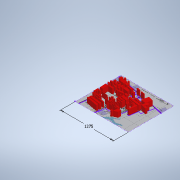
# Autodesk Inventor part: Ceg Model
Saved by Autodesk Inventor 2021 (Build 250183000, 183)
## iProperties
Created: 2021-08-03
Part Number: Ceg Model
Material: Generic
Document SubType Name: Modeling
Designer: techv
Density: 1 g/cm^3
Appearance: Default
Author: techv
Autodesk Inventor part; units mm, degrees
(part 1 of 2)
ref_plane "YZ Plane" through (0, 0, 0) normal (1, 0, 0) x (0, 1, 0)
ref_plane "XZ Plane" through (0, 0, 0) normal (0, 1, 0) x (-1, 0, 0)
ref_plane "XY Plane" through (0, 0, 0) normal (0, 0, 1) x (1, 0, 0)
sketch "Sketch1" plane through (0, 0, 0) normal (0, 1, 0) x (-1, 0, 0)
  line L0 (-1278471.3795, 0) -> (-3471.3795, 0) construction
  line L1 (-3471.3795, 0) -> (-3471.3795, -1090759.1919) construction
  line L2 (-3471.3795, -1090759.1919) -> (-1278471.3795, -1090759.1919) construction
  line L3 (-1278471.3795, -1090759.1919) -> (-1278471.3795, 0) construction
  line L4 (-570011.4545, -254930.8304) -> (-652781.9547, -243920.9646)
  line L5 (-652781.9547, -243920.9646) -> (-652781.9547, -234636.5388)
  line L6 (-652781.9547, -234636.5388) -> (-568797.9413, -245807.8223)
  line L7 (-568797.9413, -245807.8223) -> (-570011.4545, -254930.8304)
  line L8 (-501436.1788, -258320.5511) -> (-531092.2717, -254512.687)
  line L9 (-531092.2717, -254512.687) -> (-531551.829, -258091.7732)
  line L10 (-531551.829, -258091.7732) -> (-537674.5373, -257305.613)
  line L11 (-537674.5373, -257305.613) -> (-537674.5373, -262132.416)
  line L12 (-537674.5373, -262132.416) -> (-543243.6303, -262132.416)
  line L13 (-543243.6303, -262132.416) -> (-543243.6303, -255750.9615)
  line L14 (-543243.6303, -255750.9615) -> (-544918.8797, -255750.9615)
  line L15 (-544918.8797, -255750.9615) -> (-544918.8797, -248261.3499)
  line L16 (-544918.8797, -248261.3499) -> (-551485.4294, -248110.677)
  line L17 (-551485.4294, -248110.677) -> (-551473.9, -247608.2101)
  line L18 (-551473.9, -247608.2101) -> (-563231.7702, -247338.4195)
  line L19 (-563231.7702, -247338.4195) -> (-563178.5874, -245020.6323)
  line L20 (-563178.5874, -245020.6323) -> (-565590.3117, -244965.294)
  line L21 (-565590.3117, -244965.294) -> (-565542.041, -242861.5863)
  line L22 (-565542.041, -242861.5863) -> (-567752.7884, -242810.8595)
  line L23 (-567752.7884, -242810.8595) -> (-567622.1285, -237116.51)
  line L24 (-567622.1285, -237116.51) -> (-565411.3812, -237167.2367)
  line L25 (-565411.3812, -237167.2367) -> (-565358.3685, -234856.8655)
  line L26 (-565358.3685, -234856.8655) -> (-559798.004, -234984.451)
  line L27 (-559798.004, -234984.451) -> (-559904.8178, -239639.5544)
  line L28 (-559904.8178, -239639.5544) -> (-558119.111, -239680.5284)
  line L29 (-558119.111, -239680.5284) -> (-558038.8035, -236180.6106)
  line L30 (-558038.8035, -236180.6106) -> (-549698.723, -236371.9782)
  line L31 (-549698.723, -236371.9782) -> (-549769.374, -239451.0531)
  line L32 (-549769.374, -239451.0531) -> (-547223.665, -239509.4657)
  line L33 (-547223.665, -239509.4657) -> (-547179.5203, -237585.5765)
  line L34 (-547179.5203, -237585.5765) -> (-540070.8135, -237748.6895)
  line L35 (-540070.8135, -237748.6895) -> (-540175.7779, -242323.193)
  line L36 (-540175.7779, -242323.193) -> (-536543.1178, -242406.5463)
  line L37 (-536543.1178, -242406.5463) -> (-536455.3851, -238583.0282)
  line L38 (-536455.3851, -238583.0282) -> (-529068.6548, -238752.5206)
  line L39 (-529068.6548, -238752.5206) -> (-529283.5365, -248117.3798)
  line L40 (-529283.5365, -248117.3798) -> (-523156.9583, -248257.9574)
  line L41 (-523156.9583, -248257.9574) -> (-523160.4206, -248408.8486)
  line L42 (-523160.4206, -248408.8486) -> (-520279.7498, -248474.9471)
  line L43 (-520279.7498, -248474.9471) -> (-520276.2876, -248324.0559)
  line L44 (-520276.2876, -248324.0559) -> (-515159.0607, -248441.4734)
  line L45 (-515159.0607, -248441.4734) -> (-515162.523, -248592.3646)
  line L46 (-515162.523, -248592.3646) -> (-511493.6444, -248676.5489)
  line L47 (-511493.6444, -248676.5489) -> (-511460.6396, -247238.1505)
  line L48 (-511460.6396, -247238.1505) -> (-506111.3606, -247360.8925)
  line L49 (-506111.3606, -247360.8925) -> (-506184.1973, -250535.222)
  line L50 (-506184.1973, -250535.222) -> (-502834.5802, -250612.0808)
  line L51 (-502834.5802, -250612.0808) -> (-502802.8154, -249227.7254)
  line L52 (-502802.8154, -249227.7254) -> (-500231.0639, -248934.9748)
  line L53 (-500231.0639, -248934.9748) -> (-501436.1788, -258320.5511)
  line L54 (-576349.5369, -265725.8408) -> (-577610.4495, -275545.9764)
  line L55 (-577610.4495, -275545.9764) -> (-595485.6185, -273250.7916)
  line L56 (-595485.6185, -273250.7916) -> (-594224.7059, -263430.656)
  line L57 (-594224.7059, -263430.656) -> (-576349.5369, -265725.8408)
  line L58 (-597752.8257, -282598.7633) -> (-597752.8257, -289740.4021)
  line L59 (-597752.8257, -289740.4021) -> (-659285.223, -281555.5604)
  line L60 (-659285.223, -281555.5604) -> (-658213.7148, -273500.1243)
  line L61 (-658213.7148, -273500.1243) -> (-597752.8257, -282598.7633)
  line L62 (-588407.1367, -284005.1774) -> (-560547.8281, -288197.6694)
  line L63 (-560547.8281, -288197.6694) -> (-561772.7668, -296337.445)
  line L64 (-561772.7668, -296337.445) -> (-589632.0754, -292144.953)
  line L65 (-589632.0754, -292144.953) -> (-588407.1367, -284005.1774)
  line L66 (-550874.8329, -287628.5774) -> (-504335.8288, -294632.1396)
  line L67 (-504335.8288, -294632.1396) -> (-505858.7221, -304751.8384)
  line L68 (-505858.7221, -304751.8384) -> (-556890.3061, -294443.289)
  line L69 (-556890.3061, -294443.289) -> (-555803.6318, -289063.8019)
  line L70 (-555803.6318, -289063.8019) -> (-551346.6228, -289964.1325)
  line L71 (-551346.6228, -289964.1325) -> (-550874.8329, -287628.5774)
  line L72 (-537954.1525, -303901.5137) -> (-507803.7601, -307912.022)
  line L73 (-507803.7601, -307912.022) -> (-512007.3574, -328721.5677)
  line L74 (-512007.3574, -328721.5677) -> (-542054.481, -324199.8358)
  line L75 (-542054.481, -324199.8358) -> (-537954.1525, -303901.5137)
  line L76 (-583430.1694, -320870.6385) -> (-584881.4201, -332173.1501)
  line L77 (-584881.4201, -332173.1501) -> (-517286.6373, -341164.3908)
  line L78 (-517286.6373, -341164.3908) -> (-516075.1733, -332056.7879)
  line L79 (-516075.1733, -332056.7879) -> (-583430.1694, -320870.6385)
  line L80 (-615479.3563, -317270.9283) -> (-616778.3897, -327387.9534)
  line L81 (-616778.3897, -327387.9534) -> (-619540.8546, -327033.2509)
  line L82 (-619540.8546, -327033.2509) -> (-619954.6511, -323398.1367)
  line L83 (-619954.6511, -323398.1367) -> (-620991.8325, -323264.9618)
  line L84 (-620991.8325, -323264.9618) -> (-621421.5673, -326611.7868)
  line L85 (-621421.5673, -326611.7868) -> (-666953.9649, -320945.3727)
  line L86 (-666953.9649, -320945.3727) -> (-667306.5517, -323778.5798)
  line L87 (-667306.5517, -323778.5798) -> (-673124.4835, -323429.068)
  line L88 (-673124.4835, -323429.068) -> (-672710.6659, -320206.2081)
  line L89 (-672710.6659, -320206.2081) -> (-675988.6745, -319821.0215)
  line L90 (-675988.6745, -319821.0215) -> (-675583.5908, -317815.6897)
  line L91 (-675583.5908, -317815.6897) -> (-680952.2853, -318818.3556)
  line L92 (-680952.2853, -318818.3556) -> (-681544.412, -308788.1485)
  line L93 (-681544.412, -308788.1485) -> (-674349.6702, -309711.9587)
  line L94 (-674349.6702, -309711.9587) -> (-674784.0486, -302353.8958)
  line L95 (-674784.0486, -302353.8958) -> (-672818.2553, -297785.1191)
  line L96 (-672818.2553, -297785.1191) -> (-660162.9373, -299410.0712)
  line L97 (-660162.9373, -299410.0712) -> (-659745.0482, -306488.8164)
  line L98 (-659745.0482, -306488.8164) -> (-665283.6035, -307523.2057)
  line L99 (-665283.6035, -307523.2057) -> (-664969.5974, -312842.2467)
  line L100 (-664969.5974, -312842.2467) -> (-619892.3071, -318807.1617)
  line L101 (-619892.3071, -318807.1617) -> (-619413.0561, -315185.4277)
  line L102 (-619413.0561, -315185.4277) -> (-615096.7177, -314379.3015)
  line L103 (-615096.7177, -314379.3015) -> (-615479.3563, -317270.9283)
  line L104 (-553111.0094, -338765.2265) -> (-554390.9798, -348438.0549)
  line L105 (-554390.9798, -348438.0549) -> (-543302.4793, -349905.3561)
  line L106 (-543302.4793, -349905.3561) -> (-543597.3632, -352133.8147)
  line L107 (-543597.3632, -352133.8147) -> (-546543.45, -351743.9697)
  line L108 (-546543.45, -351743.9697) -> (-546081.0623, -359576.4898)
  line L109 (-546081.0623, -359576.4898) -> (-520146.7572, -363008.2827)
  line L110 (-520146.7572, -363008.2827) -> (-519136.1015, -355370.6851)
  line L111 (-519136.1015, -355370.6851) -> (-516241.938, -355753.6593)
  line L112 (-516241.938, -355753.6593) -> (-515620.402, -351056.6669)
  line L113 (-520141.6113, -351017.125) -> (-520395.6006, -352936.5406)
  line L114 (-520395.6006, -352936.5406) -> (-527923.4669, -351940.4052)
  line L115 (-527923.4669, -351940.4052) -> (-527470.3563, -348516.2159)
  line L116 (-527470.3563, -348516.2159) -> (-510967.6003, -348516.2159)
  line L117 (-510967.6003, -348516.2159) -> (-510967.6003, -345784.4652)
  line L118 (-510967.6003, -345784.4652) -> (-519303.2331, -344681.441)
  line L119 (-519303.2331, -344681.441) -> (-519487.5459, -341559.3135)
  line L120 (-519487.5459, -341559.3135) -> (-535415.6281, -341559.3135)
  line L121 (-535415.6281, -341559.3135) -> (-535415.6281, -342503.0733)
  line L122 (-535415.6281, -342503.0733) -> (-539613.4075, -342503.0733)
  line L123 (-539613.4075, -342503.0733) -> (-541104.4493, -345968.4615)
  line L124 (-541104.4493, -345968.4615) -> (-542552.2432, -344235.7674)
  line L125 (-542552.2432, -344235.7674) -> (-541828.3462, -338765.2265)
  line L126 (-541828.3462, -338765.2265) -> (-553111.0094, -338765.2265)
  line L127 (-476585.426, -56066.5539) -> (-489741.4432, -153366.8766)
  line L128 (-489741.4432, -153366.8766) -> (-517295.2524, -153366.8766)
  line L129 (-517295.2524, -153366.8766) -> (-517765.3757, -156919.6324)
  line L130 (-517765.3757, -156919.6324) -> (-645592.246, -132294.2389)
  line L131 (-645592.246, -132294.2389) -> (-624432.1327, -56065.8999)
  line L132 (-624432.1327, -56065.8999) -> (-579457.144, -45048.4869)
  line L133 (-579457.144, -45048.4869) -> (-476612.5436, -56065.8999)
  line L134 (-476612.5436, -56065.8999) -> (-476587.0054, -56065.8999)
  line L135 (-187361.2595, -477516.8715) -> (-184395.2239, -613131.8575)
  line L136 (-184395.2239, -613131.8575) -> (-115578.4666, -613131.8575)
  line L137 (-115578.4666, -613131.8575) -> (-125580.4597, -473103.9572)
  line L138 (-125580.4597, -473103.9572) -> (-187361.2595, -477516.8715)
  line L139 (-194693.2107, -601124.2909) -> (-199469.8113, -637034.0493)
  line L140 (-199469.8113, -637034.0493) -> (-302264.4641, -631807.9358)
  line L141 (-302264.4641, -631807.9358) -> (-297487.8635, -595898.1774)
  line L142 (-297487.8635, -595898.1774) -> (-194693.2107, -601124.2909)
  line L143 (-549213.9733, -482730.0886) -> (-544589.3861, -443858.4951)
  line L144 (-544589.3861, -443858.4951) -> (-559624.2309, -440599.0363)
  line L145 (-559624.2309, -440599.0363) -> (-560325.5105, -443833.8153)
  line L146 (-560325.5105, -443833.8153) -> (-608488.8408, -438103.782)
  line L147 (-608488.8408, -438103.782) -> (-608268.9514, -436255.5194)
  line L148 (-608268.9514, -436255.5194) -> (-614816.1689, -435922.6567)
  line L149 (-614816.1689, -435922.6567) -> (-615154.2722, -431189.2105)
  line L150 (-615154.2722, -431189.2105) -> (-625072.5132, -430009.2287)
  line L151 (-625072.5132, -430009.2287) -> (-624808.324, -433707.8774)
  line L152 (-624808.324, -433707.8774) -> (-680084.9307, -427131.5715)
  line L153 (-680084.9307, -427131.5715) -> (-679654.7278, -423515.5353)
  line L154 (-679654.7278, -423515.5353) -> (-696663.7118, -421491.9617)
  line L155 (-696663.7118, -421491.9617) -> (-702453.7118, -459966.7876)
  line L156 (-702453.7118, -459966.7876) -> (-688325.8186, -463029.6251)
  line L157 (-688325.8186, -463029.6251) -> (-686234.3175, -445449.6816)
  line L158 (-686234.3175, -445449.6816) -> (-674994.9466, -446786.8393)
  line L159 (-674994.9466, -446786.8393) -> (-674278.956, -440768.6381)
  line L160 (-674278.956, -440768.6381) -> (-632338.1096, -447080.2326)
  line L161 (-632338.1096, -447080.2326) -> (-631993.6447, -451902.7415)
  line L162 (-631993.6447, -451902.7415) -> (-613386.5993, -455936.6307)
  line L163 (-613386.5993, -455936.6307) -> (-613820.147, -449866.964)
  line L164 (-570176.8772, -456434.7529) -> (-613820.147, -449866.964)
  line L165 (-570176.8772, -456434.7529) -> (-571280.212, -463766.4646)
  line L166 (-571280.212, -463766.4646) -> (-560606.0593, -465372.7966)
  line L167 (-560606.0593, -465372.7966) -> (-562717.3757, -483119.2962)
  line L168 (-562717.3757, -483119.2962) -> (-549598.6379, -485963.3552)
  line L169 (-549598.6379, -485963.3552) -> (-549231.796, -482723.5649)
  line L170 (-549231.796, -482723.5649) -> (-549213.4568, -482725.7467)
  line L171 (-591998.5121, -485963.3552) -> (-594855.1622, -509974.6964)
  line L172 (-594855.1622, -509974.6964) -> (-552882.8577, -514968.1779)
  line L173 (-552882.8577, -514968.1779) -> (-552705.3423, -513400.4382)
  line L174 (-552705.3423, -513400.4382) -> (-544850.7477, -512839.3958)
  line L175 (-544850.7477, -512839.3958) -> (-545055.3691, -509974.6964)
  line L176 (-545055.3691, -509974.6964) -> (-532080.6056, -511927.2427)
  line L177 (-532080.6056, -511927.2427) -> (-530643.8391, -499850.6182)
  line L178 (-530643.8391, -499850.6182) -> (-543305.1328, -498344.293)
  line L179 (-543305.1328, -498344.293) -> (-591998.5121, -485963.3552)
  line L180 (-602714.2054, -471056.9767) -> (-606522.915, -503070.7766)
  line L181 (-606522.915, -503070.7766) -> (-613820.147, -503592.0074)
  line L182 (-613820.147, -503592.0074) -> (-614304.2178, -507660.8253)
  line L183 (-614304.2178, -507660.8253) -> (-620991.8325, -506865.194)
  line L184 (-620991.8325, -506865.194) -> (-660296.0332, -498344.293)
  line L185 (-660296.0332, -498344.293) -> (-657354.4584, -484775.7458)
  line L186 (-657354.4584, -484775.7458) -> (-642875.9082, -486498.2715)
  line L187 (-602714.2054, -471056.9767) -> (-608875.3257, -471056.9767)
  line L188 (-608875.3257, -471056.9767) -> (-608875.3257, -475461.8252)
  line L189 (-608875.3257, -475461.8252) -> (-655671.1861, -469894.4811)
  line L190 (-655671.1861, -469894.4811) -> (-656680.2012, -478375.6763)
  line L191 (-656680.2012, -478375.6763) -> (-638246.024, -480568.8064)
  line L192 (-638246.024, -480568.8064) -> (-639006.2293, -486958.6505)
  line L193 (-639006.2293, -486958.6505) -> (-642875.9082, -486498.2715)
  line L194 (-552532.2534, -349791.3441) -> (-555407.2659, -373957.0294)
  line L195 (-555407.2659, -373957.0294) -> (-565999.2567, -372696.8911)
  line L196 (-565999.2567, -372696.8911) -> (-569455.0267, -401744.0858)
  line L197 (-569455.0267, -401744.0858) -> (-567727.1417, -401949.6537)
  line L198 (-567727.1417, -401949.6537) -> (-568639.4398, -409617.9014)
  line L199 (-568639.4398, -409617.9014) -> (-589632.0754, -405783.7776)
  line L200 (-552532.2534, -349791.3441) -> (-589632.0754, -345377.5461)
  line L201 (-589632.0754, -345377.5461) -> (-596221.5242, -369101.3217)
  line L202 (-596221.5242, -369101.3217) -> (-573957.1769, -371750.1304)
  line L203 (-573957.1769, -371750.1304) -> (-574364.3175, -375172.3177)
  line L204 (-574364.3175, -375172.3177) -> (-592926.7998, -377410.142)
  line L205 (-592926.7998, -377410.142) -> (-596530.5104, -407700.8395)
  line L206 (-596530.5104, -407700.8395) -> (-590121.4722, -408463.3283)
  line L207 (-590121.4722, -408463.3283) -> (-589656.3149, -404553.4868)
  line L208 (-612582.1275, -354699.6255) -> (-614276.5325, -363927.9404)
  line L209 (-614276.5325, -363927.9404) -> (-653224.0488, -359809.8605)
  line L210 (-653224.0488, -359809.8605) -> (-653661.6547, -363948.6009)
  line L211 (-653661.6547, -363948.6009) -> (-662437.7472, -362337.2281)
  line L212 (-662437.7472, -362337.2281) -> (-661807.0701, -358902.3427)
  line L213 (-661807.0701, -358902.3427) -> (-686257.2938, -356317.1207)
  line L214 (-686257.2938, -356317.1207) -> (-685006.7827, -344490.1763)
  line L215 (-685006.7827, -344490.1763) -> (-661757.6983, -348758.9259)
  line L216 (-661757.6983, -348758.9259) -> (-660529.2194, -351942.7266)
  line L217 (-660529.2194, -351942.7266) -> (-659183.6861, -344614.4876)
  line L218 (-659183.6861, -344614.4876) -> (-651761.4731, -345977.2754)
  line L219 (-651761.4731, -345977.2754) -> (-652240.3559, -350506.3991)
  line L220 (-612582.1275, -354699.6255) -> (-652240.3559, -350506.3991)
  line L221 (-619040.8686, -391036.3643) -> (-622253.4844, -408533.3791)
  line L222 (-622253.4844, -408533.3791) -> (-654740.2355, -404629.4015)
  line L223 (-654740.2355, -404629.4015) -> (-655210.0865, -408539.243)
  line L224 (-655210.0865, -408539.243) -> (-661039.7209, -407838.6878)
  line L225 (-661039.7209, -407838.6878) -> (-660569.8699, -403928.8462)
  line L226 (-660569.8699, -403928.8462) -> (-661039.7209, -403872.3836)
  line L227 (-661039.7209, -403872.3836) -> (-663153.8905, -403618.3209)
  line L228 (-663153.8905, -403618.3209) -> (-662099.9972, -397878.4539)
  line L229 (-662099.9972, -397878.4539) -> (-690293.5105, -394490.4006)
  line L230 (-690293.5105, -394490.4006) -> (-691116.8059, -383339.0769)
  line L231 (-691116.8059, -383339.0769) -> (-659282.3949, -387164.662)
  line L232 (-659282.3949, -387164.662) -> (-658199.8265, -389970.312)
  line L233 (-658199.8265, -389970.312) -> (-624423.9703, -394490.4006)
  line L234 (-624423.9703, -394490.4006) -> (-624010.8351, -391403.2939)
  line L235 (-624010.8351, -391403.2939) -> (-619040.8686, -391036.3643)
  line L236 (-525546.2206, -366271.6801) -> (-527000.3094, -377137.1961)
  line L237 (-527000.3094, -377137.1961) -> (-542381.0654, -375078.8506)
  line L238 (-542381.0654, -375078.8506) -> (-540294.7007, -363715.7882)
  line L239 (-540294.7007, -363715.7882) -> (-525976.7636, -365631.9008)
  line L240 (-525546.2206, -366271.6801) -> (-525976.7636, -365631.9008)
  line L241 (-530283.2794, -380783.8087) -> (-530283.2794, -387807.8656)
  line L242 (-530283.2794, -387807.8656) -> (-523324.7323, -396698.5123)
  line L243 (-523324.7323, -396698.5123) -> (-531835.9847, -402426.2061)
  line L244 (-531835.9847, -402426.2061) -> (-525274.8769, -405206.3339)
  line L245 (-525274.8769, -405206.3339) -> (-527295.3343, -415108.5874)
  line L246 (-527295.3343, -415108.5874) -> (-537411.5471, -413977.7521)
  line L247 (-537411.5471, -413977.7521) -> (-537960.7439, -418890.75)
  line L248 (-537960.7439, -418890.75) -> (-542012.3194, -418890.75)
  line L249 (-542012.3194, -418890.75) -> (-542012.3194, -413463.4573)
  line L250 (-542012.3194, -413463.4573) -> (-557798.1762, -411511.6039)
  line L251 (-557798.1762, -411511.6039) -> (-556372.7765, -399983.5067)
  line L252 (-556372.7765, -399983.5067) -> (-543751.1927, -401544.1113)
  line L253 (-543751.1927, -401544.1113) -> (-550092.0743, -392121.6726)
  line L254 (-550092.0743, -392121.6726) -> (-557798.7052, -392121.6726)
  line L255 (-557798.7052, -392121.6726) -> (-557798.7052, -380669.7544)
  line L256 (-557798.7052, -380669.7544) -> (-550107.5725, -382239.0543)
  line L257 (-550107.5725, -382239.0543) -> (-551651.274, -389804.7292)
  line L258 (-551651.274, -389804.7292) -> (-550137.1393, -390113.6735)
  line L259 (-550137.1393, -390113.6735) -> (-548593.4378, -382547.9986)
  line L260 (-548593.4378, -382547.9986) -> (-542012.3194, -383890.811)
  line L261 (-542012.3194, -378390.6135) -> (-530283.2794, -380783.8087)
  line L262 (-542012.3194, -378390.6135) -> (-542012.3194, -383890.811)
  line L263 (-669472.0303, -502604.6558) -> (-667984.8054, -484775.8335)
  line L264 (-667984.8054, -484775.8335) -> (-678048.3541, -482722.4655)
  line L265 (-678048.3541, -482722.4655) -> (-678048.3541, -472750.6156)
  line L266 (-678048.3541, -472750.6156) -> (-697343.5605, -470364.8462)
  line L267 (-697343.5605, -470364.8462) -> (-700714.7328, -497873.828)
  line L268 (-700714.7328, -497873.828) -> (-669472.0303, -502604.6558)
  line L269 (-700585.7729, -569956.4652) -> (-647479.6407, -577997.894)
  line L270 (-647479.6407, -577997.894) -> (-647479.6407, -596442.1119)
  line L271 (-647479.6407, -596442.1119) -> (-641279.3144, -596442.1119)
  line L272 (-641279.3144, -596442.1119) -> (-638688.0358, -579329.1351)
  line L273 (-638688.0358, -579329.1351) -> (-584126.5188, -587590.9409)
  line L274 (-584126.5188, -587590.9409) -> (-587303.3697, -603160.6742)
  line L275 (-587303.3697, -603160.6742) -> (-573577.8574, -605961.2299)
  line L276 (-573577.8574, -605961.2299) -> (-562737.8601, -552834.4464)
  line L277 (-562737.8601, -552834.4464) -> (-557798.7052, -534594.0161)
  line L278 (-557798.7052, -534594.0161) -> (-562862.0396, -533222.9633)
  line L279 (-562862.0396, -533222.9633) -> (-563391.429, -536719.0862)
  line L280 (-563391.429, -536719.0862) -> (-585101.8473, -533431.6545)
  line L281 (-585101.8473, -533431.6545) -> (-585704.808, -529064.0055)
  line L282 (-585704.808, -529064.0055) -> (-597126.2339, -529064.0055)
  line L283 (-597126.2339, -529064.0055) -> (-598304.3443, -536844.3253)
  line L284 (-598304.3443, -536844.3253) -> (-605458.486, -537261.4873)
  line L285 (-605458.486, -537261.4873) -> (-604889.078, -530435.4354)
  line L286 (-604889.078, -530435.4354) -> (-624023.3318, -527538.0913)
  line L287 (-624023.3318, -527538.0913) -> (-624431.7444, -520533.9978)
  line L288 (-624431.7444, -520533.9978) -> (-641323.4982, -519124.9402)
  line L289 (-641323.4982, -519124.9402) -> (-641800.7481, -524846.2021)
  line L290 (-641800.7481, -524846.2021) -> (-661568.7166, -521852.8997)
  line L291 (-661568.7166, -521852.8997) -> (-663975.6196, -527533.1963)
  line L292 (-663975.6196, -527533.1963) -> (-671456.9934, -526400.3528)
  line L293 (-671456.9934, -526400.3528) -> (-670756.7425, -518005.7591)
  line L294 (-670756.7425, -518005.7591) -> (-680558.4164, -517188.1339)
  line L295 (-680558.4164, -517188.1339) -> (-682728.9156, -518648.7832)
  line L296 (-682728.9156, -518648.7832) -> (-704824.703, -515302.9982)
  line L297 (-704824.703, -515302.9982) -> (-706568.8487, -513074.5757)
  line L298 (-706568.8487, -513074.5757) -> (-710355.1521, -512501.2466)
  line L299 (-710355.1521, -512501.2466) -> (-711609.5539, -527538.9895)
  line L300 (-711609.5539, -527538.9895) -> (-708010.5127, -529064.0055)
  line L301 (-708010.5127, -529064.0055) -> (-716307.4983, -583857.8522)
  line L302 (-716307.4983, -583857.8522) -> (-702995.9612, -585873.5097)
  line L303 (-702995.9612, -585873.5097) -> (-700585.7729, -569956.4652)
  line L304 (-678048.3541, -605417.4517) -> (-685898.1685, -643985.6091)
  line L305 (-685898.1685, -643985.6091) -> (-744585.6764, -632040.8837)
  line L306 (-744585.6764, -632040.8837) -> (-737322.0974, -596442.1119)
  line L307 (-737322.0974, -596442.1119) -> (-678048.3541, -605417.4517)
  line L308 (-613167.9866, -615241.757) -> (-620841.7228, -652850.7072)
  line L309 (-620841.7228, -652850.7072) -> (-557798.7052, -665714.0144)
  line L310 (-557798.7052, -665714.0144) -> (-551568.4914, -624569.2665)
  line L311 (-551568.4914, -624569.2665) -> (-613167.9866, -615241.757)
  line L312 (-612786.93, -752159.811) -> (-621282.3669, -793795.9132)
  line L313 (-621282.3669, -793795.9132) -> (-650128.5786, -787910.1277)
  line L314 (-650128.5786, -787910.1277) -> (-641933.5601, -747746.3744)
  line L315 (-641933.5601, -747746.3744) -> (-612786.93, -752159.811)
  line L316 (-586513.7316, -891682.02) -> (-588388.1453, -914152.4534)
  line L317 (-588388.1453, -914152.4534) -> (-663973.0845, -898730.0905)
  line L318 (-663973.0845, -898730.0905) -> (-662098.6708, -876259.6571)
  line L319 (-662098.6708, -876259.6571) -> (-586513.7316, -891682.02)
  line L320 (-794290.5179, -854445.9199) -> (-797756.5425, -871432.8927)
  line L321 (-797756.5425, -871432.8927) -> (-714783.3657, -886402.2791)
  line L322 (-714783.3657, -886402.2791) -> (-713099.0778, -866211.0701)
  line L323 (-713099.0778, -866211.0701) -> (-794290.5179, -854445.9199)
  line L324 (-991429.2904, -686586.4577) -> (-1024430.5176, -833332.1314)
  line L325 (-1024430.5176, -833332.1314) -> (-912287.5284, -858551.657)
  line L326 (-912287.5284, -858551.657) -> (-879286.3013, -711805.9832)
  line L327 (-879286.3013, -711805.9832) -> (-991429.2904, -686586.4577)
  line L328 (-984910.363, -615769.2318) -> (-1009672.0216, -725876.2363)
  line L329 (-1009672.0216, -725876.2363) -> (-1069553.4131, -709661.5164)
  line L330 (-1069553.4131, -709661.5164) -> (-1058486.6277, -660451.138)
  line L331 (-1058486.6277, -660451.138) -> (-1048021.2027, -662804.6783)
  line L332 (-1048021.2027, -662804.6783) -> (-1035036.6843, -605066.7679)
  line L333 (-1035036.6843, -605066.7679) -> (-1053789.5413, -600849.49)
  line L334 (-1053789.5413, -600849.49) -> (-1062793.1781, -634100.1602)
  line L335 (-1062793.1781, -634100.1602) -> (-1114026.1729, -622578.5143)
  line L336 (-1114026.1729, -622578.5143) -> (-1104052.69, -578229.6944)
  line L337 (-1104052.69, -578229.6944) -> (-982610.0716, -605540.5877)
  line L338 (-982610.0716, -605540.5877) -> (-984910.363, -615769.2318)
  line L339 (-932650.133, -347466.5066) -> (-958974.5483, -542270.8246)
  line L340 (-958974.5483, -542270.8246) -> (-923329.2267, -545244.2465)
  line L341 (-923329.2267, -545244.2465) -> (-922968.203, -540916.3026)
  line L342 (-922968.203, -540916.3026) -> (-892345.0705, -540919.9176)
  line L343 (-892340.3799, -501185.1888) -> (-916798.1218, -497481.7522)
  line L344 (-916798.1218, -497481.7522) -> (-900153.2271, -361658.3465)
  line L345 (-900153.2271, -361658.3465) -> (-934007.2821, -357509.5978)
  line L346 (-892340.3799, -501185.1888) -> (-892345.0705, -540919.9176)
  line L347 (-835964.5512, -559580.7768) -> (-829965.7375, -510630.0725)
  line L348 (-829965.7375, -510630.0725) -> (-860041.1469, -506075.9984)
  line L349 (-860041.1469, -506075.9984) -> (-862720.5659, -517990.4989)
  line L350 (-862720.5659, -517990.4989) -> (-843497.1712, -522313.5948)
  line L351 (-843497.1712, -522313.5948) -> (-838195.2734, -529087.6094)
  line L352 (-838195.2734, -529087.6094) -> (-863967.4685, -529064.0055)
  line L353 (-863967.4685, -529064.0055) -> (-876882.4121, -559543.3016)
  line L354 (-876882.4121, -559543.3016) -> (-835964.5512, -559580.7768)
  line L355 (-870476.811, -430215.5837) -> (-870504.2826, -460210.7794)
  line L356 (-870504.2826, -460210.7794) -> (-829953.9, -466350.9933)
  line L357 (-829953.9, -466350.9933) -> (-831723.3058, -478036.2675)
  line L358 (-831723.3058, -478036.2675) -> (-892336.7704, -470608.2051)
  line L359 (-892336.7704, -470608.2051) -> (-892338.4628, -484944.997)
  line L360 (-828011.7569, -494685.4658) -> (-818085.847, -439667.561)
  line L361 (-818085.847, -439667.561) -> (-870476.811, -430215.5837)
  line L362 (-795379.4654, -447319.1215) -> (-799325.8119, -469193.1581)
  line L363 (-799325.8119, -469193.1581) -> (-754718.4125, -477240.8841)
  line L364 (-754718.4125, -477240.8841) -> (-755134.0424, -451024.8444)
  line L365 (-795379.4654, -447319.1215) -> (-755134.0424, -451024.8444)
  line L366 (-755134.0424, -487422.133) -> (-756851.6553, -506075.9984)
  line L367 (-756851.6553, -506075.9984) -> (-805177.1475, -501626.2778)
  line L368 (-805177.1475, -501626.2778) -> (-802931.7862, -477240.8841)
  line L369 (-802931.7862, -477240.8841) -> (-755134.0424, -487422.133)
  line L370 (-754888.3671, -567182.5505) -> (-754888.3671, -554737.1107)
  line L371 (-754888.3671, -554737.1107) -> (-764815.2517, -554737.1107)
  line L372 (-764815.2517, -554737.1107) -> (-764815.2517, -559478.3612)
  line L373 (-764815.2517, -559478.3612) -> (-802802.9194, -554874.5981)
  line L374 (-802802.9194, -554874.5981) -> (-801640.6922, -545284.5522)
  line L375 (-801640.6922, -545284.5522) -> (-816937.5647, -543430.7091)
  line L376 (-816937.5647, -543430.7091) -> (-816937.5647, -559662.7468)
  line L377 (-816937.5647, -559662.7468) -> (-754888.3671, -567182.5505)
  line L378 (-741047.3685, -508326.0673) -> (-734335.073, -452939.9745)
  line L379 (-734335.073, -452939.9745) -> (-736086.414, -452778.7143)
  line L380 (-736086.414, -452778.7143) -> (-747620.1626, -506926.0169)
  line L381 (-747620.1626, -506926.0169) -> (-741047.3685, -508326.0673)
  line L382 (-744221.5271, -545379.596) -> (-764815.2517, -540992.9907)
  line L383 (-764815.2517, -540992.9907) -> (-764815.2517, -540992.9907)
  line L384 (-764815.2517, -540992.9907) -> (-788987.2583, -529064.0055)
  line L385 (-788987.2583, -529064.0055) -> (-790368.8003, -535549.9087)
  line L386 (-790368.8003, -535549.9087) -> (-789678.0293, -532306.9571)
  line L387 (-789678.0293, -528723.1072) -> (-807520.894, -527080.1697)
  line L388 (-807520.894, -527080.1697) -> (-807672.1726, -528723.1072)
  line L389 (-807672.1726, -528723.1072) -> (-798332.8989, -517990.4989)
  line L390 (-798332.8989, -517990.4989) -> (-798594.9645, -520152.9176)
  line L391 (-798594.9645, -520152.9176) -> (-798332.8989, -517990.4989)
  line L392 (-798332.8989, -517990.4989) -> (-797440.8815, -510630.0725)
  line L393 (-797440.8815, -510630.0725) -> (-760000.7759, -514077.4871)
  line L394 (-760000.7759, -514077.4871) -> (-757035.0764, -508068.0147)
  line L395 (-757035.0764, -508068.0147) -> (-736086.414, -509996.9282)
  line L396 (-736086.414, -509996.9282) -> (-737156.1717, -521614.865)
  line L397 (-737156.1717, -521614.865) -> (-747630.503, -520650.4083)
  line L398 (-747630.503, -520650.4083) -> (-747630.503, -532594.7644)
  line L399 (-747630.503, -532594.7644) -> (-738246.7394, -533458.8037)
  line L400 (-744618.1723, -545295.1078) -> (-738246.7394, -533458.8037)
  line L401 (-698438.2408, -301694.6282) -> (-696913.26, -269545.9789)
  line L402 (-696913.26, -269545.9789) -> (-772917.1558, -260130.4689)
  line L403 (-772917.1558, -260130.4689) -> (-777163.1226, -294404.7696)
  line L404 (-777163.1226, -294404.7696) -> (-698438.2408, -301694.6282)
  line L405 (-696238.5559, -255322.3094) -> (-771040.4294, -244981.1552)
  line L406 (-771040.4294, -244981.1552) -> (-770163.8659, -237905.3579)
  line L407 (-770163.8659, -237905.3579) -> (-695580.1989, -241443.2565)
  line L408 (-695580.1989, -241443.2565) -> (-696238.5559, -255322.3094)
  line L409 (-208111.8327, -815173.3425) -> (-206014.2925, -798241.575)
  line L410 (-206014.2925, -798241.575) -> (-299365.4284, -782304.919)
  line L411 (-299365.4284, -782304.919) -> (-302807.1111, -802465.0449)
  line L412 (-302807.1111, -802465.0449) -> (-291309.6368, -804427.863)
  line L413 (-291309.6368, -804427.863) -> (-289420.2086, -793360.2793)
  line L414 (-289420.2086, -793360.2793) -> (-280051.7753, -794959.6332)
  line L415 (-280051.7753, -794959.6332) -> (-281941.2036, -806027.2168)
  line L416 (-281941.2036, -806027.2168) -> (-208111.8327, -815173.3425)
  line L417 (-283239.372, -766144.7304) -> (-281420.2142, -746499.2213)
  line L418 (-281420.2142, -746499.2213) -> (-291553.8062, -745560.8591)
  line L419 (-291553.8062, -745560.8591) -> (-288211.017, -725980.0155)
  line L420 (-288211.017, -725980.0155) -> (-320276.4134, -723010.7865)
  line L421 (-320276.4134, -723010.7865) -> (-328778.0191, -772810.101)
  line L422 (-328778.0191, -772810.101) -> (-293842.9671, -778774.1196)
  line L423 (-293842.9671, -778774.1196) -> (-283239.372, -766144.7304)
  line L424 (-227780.3781, -928893.9269) -> (-337439.7206, -914655.0929)
  line L425 (-337439.7206, -914655.0929) -> (-327221.2593, -835958.3578)
  line L426 (-327221.2593, -835958.3578) -> (-215771.734, -858551.657)
  line L427 (-215771.734, -858551.657) -> (-227780.3781, -928893.9269)
  line L428 (-356535.6255, -898962.3672) -> (-346781.5426, -841826.4967)
  line L429 (-346781.5426, -841826.4967) -> (-402311.6048, -832346.5531)
  line L430 (-402311.6048, -832346.5531) -> (-412065.6877, -889482.4236)
  line L431 (-412065.6877, -889482.4236) -> (-389961.5726, -893255.979)
  line L432 (-389961.5726, -893255.979) -> (-389961.5726, -905438.6963)
  line L433 (-389961.5726, -905438.6963) -> (-379725.3032, -905438.6963)
  line L434 (-379725.3032, -905438.6963) -> (-377994.2818, -895299.0028)
  line L435 (-377994.2818, -895299.0028) -> (-356535.6255, -898962.3672)
  line L436 (-161762.5899, -961065.5244) -> (-152577.2162, -890325.0383)
  line L437 (-152577.2162, -890325.0383) -> (-196003.5869, -882911.4045)
  line L438 (-196003.5869, -882911.4045) -> (-207754.1635, -951742.0089)
  line L439 (-207754.1635, -951742.0089) -> (-164539.7553, -960502.5312)
  line L440 (-164539.7553, -960502.5312) -> (-164539.7553, -960502.5312)
  line L441 (-161762.5899, -961065.5244) -> (-164539.7553, -960502.5312)
  line L442 (-221776.056, -983667.832) -> (-264481.195, -967642.3551)
  line L443 (-264481.195, -967642.3551) -> (-261169.9648, -940913.4372)
  line L444 (-261169.9648, -940913.4372) -> (-227968.2827, -945026.526)
  line L445 (-227968.2827, -945026.526) -> (-228976.0328, -953161.288)
  line L446 (-228976.0328, -953161.288) -> (-219805.8494, -967763.927)
  line L447 (-219805.8494, -967763.927) -> (-221776.056, -983667.832)
  line L448 (-332330.4899, -953824.1563) -> (-332330.4899, -926487.615)
  line L449 (-332330.4899, -926487.615) -> (-356742.7346, -917326.7067)
  line L450 (-356742.7346, -917326.7067) -> (-360826.7843, -950293.98)
  line L451 (-360826.7843, -950293.98) -> (-332330.4899, -953824.1563)
  line L452 (-529280.8888, -626886.3607) -> (-421798.5365, -610302.1273)
  line L453 (-421798.5365, -610302.1273) -> (-421798.5365, -624482.2684)
  line L454 (-421798.5365, -624482.2684) -> (-422866.6508, -646780.0306)
  line L455 (-422866.6508, -646780.0306) -> (-462908.2342, -644861.9463)
  line L456 (-462908.2342, -644861.9463) -> (-463165.2155, -650226.6415)
  line L457 (-463165.2155, -650226.6415) -> (-486010.1119, -653751.5466)
  line L458 (-486010.1119, -653751.5466) -> (-522453.015, -652323.8427)
  line L459 (-522453.015, -652323.8427) -> (-521723.5739, -633704.4693)
  line L460 (-521723.5739, -633704.4693) -> (-528189.8509, -633451.1434)
  line L461 (-529280.8888, -626886.3607) -> (-528189.8509, -633451.1434)
  line L462 (-367077.2832, -640137.5078) -> (-410253.9255, -634208.1964)
  line L463 (-410253.9255, -634208.1964) -> (-406959.1063, -610215.658)
  line L464 (-406959.1063, -610215.658) -> (-363782.464, -616144.9694)
  line L465 (-363782.464, -616144.9694) -> (-367077.2832, -640137.5078)
  line L466 (-431323.4373, -787634.2387) -> (-537725.812, -773022.3381)
  line L467 (-537725.812, -773022.3381) -> (-547645.2248, -713337.1604)
  line L468 (-547645.2248, -713337.1604) -> (-423462.377, -730390.797)
  line L469 (-423462.377, -730390.797) -> (-431323.4373, -787634.2387)
  line L470 (-403199.24, -782906.0088) -> (-394811.0565, -721824.11)
  line L471 (-394811.0565, -721824.11) -> (-407513.2638, -720079.7562)
  line L472 (-407513.2638, -720079.7562) -> (-415901.4472, -781161.655)
  line L473 (-415901.4472, -781161.655) -> (-403199.24, -782906.0088)
  line L474 (-344977.4106, -790901.4279) -> (-336589.2272, -729819.5292)
  line L475 (-336589.2272, -729819.5292) -> (-380285.7347, -736320.1084)
  line L476 (-386988.9332, -785132.1188) -> (-344977.4106, -790901.4279)
  line L477 (-380285.7347, -736320.1084) -> (-386988.9332, -785132.1188)
  line L478 (-204146.9874, -734612.109) -> (-207637.4564, -760029.3489)
  line L479 (-207637.4564, -760029.3489) -> (-238703.7818, -779393.1288)
  line L480 (-238703.7818, -779393.1288) -> (-251256.3216, -777669.3283)
  line L481 (-251256.3216, -777669.3283) -> (-244580.8813, -729059.4506)
  line L482 (-244580.8813, -729059.4506) -> (-204146.9874, -734612.109)
  line L483 (-143185.0905, -772664.245) -> (-150536.1437, -826193.8672)
  line L484 (-150536.1437, -826193.8672) -> (-181977.6487, -813285.6683)
  line L485 (-181977.6487, -813285.6683) -> (-177935.7028, -783852.6287)
  line L486 (-177935.7028, -783852.6287) -> (-188915.3981, -779344.9535)
  line L487 (-188915.3981, -779344.9535) -> (-186573.8427, -762293.985)
  line L488 (-186573.8427, -762293.985) -> (-175189.8102, -763857.3181)
  line L489 (-175189.8102, -763857.3181) -> (-177091.9423, -777708.4508)
  line L490 (-177091.9423, -777708.4508) -> (-143185.0905, -772664.245)
  line L491 (-112499.3961, -756681.785) -> (-173062.2822, -748364.8759)
  line L492 (-173062.2822, -748364.8759) -> (-173884.8818, -754354.9625)
  line L493 (-173884.8818, -754354.9625) -> (-184546.219, -752890.8748)
  line L494 (-184546.219, -752890.8748) -> (-179720.8947, -717753.3539)
  line L495 (-179720.8947, -717753.3539) -> (-108496.6713, -727534.3506)
  line L496 (-108496.6713, -727534.3506) -> (-111583.404, -750011.624)
  line L497 (-111583.404, -750011.624) -> (-133949.315, -746940.1843)
  line L498 (-133949.315, -746940.1843) -> (-135481.099, -758094.4795)
  line L499 (-135481.099, -758094.4795) -> (-113115.188, -761165.9192)
  line L500 (-113115.188, -761165.9192) -> (-112499.3961, -756681.785)
  line L501 (-210305.1067, -703466.2132) -> (-209100.6515, -694695.4928)
  line L502 (-209100.6515, -694695.4928) -> (-311292.3741, -654496.8675)
  line L503 (-311292.3741, -654496.8675) -> (-316023.4725, -688948.2453)
  line L504 (-316023.4725, -688948.2453) -> (-207562.862, -703842.797)
  line L505 (-207562.862, -703842.797) -> (-210305.1067, -703466.2132)
  line L506 (-335146.052, -719310.4746) -> (-330699.7289, -686932.8016)
  line L507 (-361068.5804, -682762.3435) -> (-373379.9507, -714059.9345)
  line L508 (-373379.9507, -714059.9345) -> (-335146.052, -719310.4746)
  line L509 (-330699.7289, -686932.8016) -> (-361068.5804, -682762.3435)
  line L510 (-122663.7174, -691583.4322) -> (-101771.3322, -678561.1148)
  line L511 (-101771.3322, -678561.1148) -> (-151239.4155, -646963.4702)
  line L512 (-151239.4155, -646963.4702) -> (-175137.4777, -684377.3771)
  line L513 (-175137.4777, -684377.3771) -> (-122663.7174, -691583.4322)
  line L514 (-439639.9417, -848194.1781) -> (-436024.6698, -821868.1362)
  line L515 (-436024.6698, -821868.1362) -> (-553657.1695, -798092.703)
  line L516 (-553657.1695, -798092.703) -> (-559662.9927, -841826.4967)
  line L517 (-559662.9927, -841826.4967) -> (-439639.9417, -848194.1781)
  line L518 (-221776.056, -360862.4672) -> (-368782.9045, -332220.4384)
  line L519 (-368782.9045, -332220.4384) -> (-354263.0014, -315825.1149)
  line L520 (-354263.0014, -315825.1149) -> (-354263.0014, -307523.2057)
  line L521 (-354263.0014, -307523.2057) -> (-387456.1262, -301056.0346)
  line L522 (-387456.1262, -301056.0346) -> (-388665.6043, -335402.8303)
  line L523 (-388665.6043, -335402.8303) -> (-223100.5749, -367660.636)
  line L524 (-223100.5749, -367660.636) -> (-221776.056, -360862.4672)
  line L525 (-210123.6903, -301056.0346) -> (-204751.0175, -273480.4848)
  line L526 (-204751.0175, -273480.4848) -> (-212396.8644, -269545.9789)
  line L527 (-212396.8644, -269545.9789) -> (-214081.7136, -278193.5641)
  line L528 (-214081.7136, -278193.5641) -> (-311285.3187, -269546.6066)
  line L529 (-311285.3187, -269546.6066) -> (-313026.6415, -289121.4519)
  line L530 (-313026.6415, -289121.4519) -> (-210123.6903, -301056.0346)
  line L531 (-228999.9924, -250148.9862) -> (-227968.2827, -241253.327)
  line L532 (-227968.2827, -241253.327) -> (-313082.0275, -224953.8821)
  line L533 (-313082.0275, -224953.8821) -> (-315175.0396, -235883.3401)
  line L534 (-315175.0396, -235883.3401) -> (-300120.3544, -238766.3411)
  line L535 (-300120.3544, -238766.3411) -> (-301132.9223, -250148.9862)
  line L536 (-301132.9223, -250148.9862) -> (-290219.399, -250148.9862)
  line L537 (-290219.399, -250148.9862) -> (-282634.009, -242115.0097)
  line L538 (-282634.009, -242115.0097) -> (-228999.9924, -250148.9862)
  line L539 (-329484.4717, -238769.0872) -> (-327015.371, -222285.6201)
  line L540 (-327015.371, -222285.6201) -> (-471609.0398, -200626.5648)
  line L541 (-471609.0398, -200626.5648) -> (-471609.0398, -222285.6201)
  line L542 (-471609.0398, -222285.6201) -> (-329484.4717, -238769.0872)
  line L543 (-258299.8505, -341629.8177) -> (-241980.9022, -319191.4978)
  line L544 (-241980.9022, -319191.4978) -> (-253938.2827, -304351.837)
  line L545 (-253938.2827, -304351.837) -> (-264361.4316, -312750.5166)
  line L546 (-264361.4316, -312750.5166) -> (-272053.3881, -303204.4438)
  line L547 (-272053.3881, -303204.4438) -> (-315175.0396, -301056.0346)
  line L548 (-315175.0396, -301056.0346) -> (-314138.8905, -327465.816)
  line L549 (-314138.8905, -327465.816) -> (-265881.6632, -332220.4384)
  line L550 (-265881.6632, -332220.4384) -> (-259178.1687, -340539.7843)
  line L551 (-259178.1687, -340539.7843) -> (-258299.8505, -341629.8177)
  line L552 (-190657.297, -196584.3875) -> (-464849.7765, -166413.2228)
  line L553 (-190657.297, -196584.3875) -> (-187087.2018, -155642.8934)
  line L554 (-187087.2018, -155642.8934) -> (-459094.1067, -121095.8413)
  line L555 (-459094.1067, -121095.8413) -> (-464849.7765, -166413.2228)
  line L556 (-185703.1973, -139771.2685) -> (-454436.4268, -105639.9994)
  line L557 (-454436.4268, -105639.9994) -> (-455574.3556, -55823.4238)
  line L558 (-455574.3556, -55823.4238) -> (-179720.8947, -108360.0767)
  line L559 (-179720.8947, -108360.0767) -> (-185703.1973, -139771.2685)
  line L560 (-780427.859, -242114.1157) -> (-767429.6125, -139772.1624)
  line L561 (-767429.6125, -139772.1624) -> (-850229.0913, -178373.6403)
  line L562 (-850229.0913, -178373.6403) -> (-855669.0715, -249425.8975)
  line L563 (-855669.0715, -249425.8975) -> (-780427.859, -242114.1157)
  line L564 (-701996.813, -139772.1624) -> (-755747.1621, -164830.8095)
  line L565 (-755747.1621, -164830.8095) -> (-759341.2685, -127845.9899)
  line L566 (-759341.2685, -127845.9899) -> (-728871.9875, -113641.0783)
  line L567 (-728871.9875, -113641.0783) -> (-701996.813, -139772.1624)
  line L568 (-764504.4344, -631963.1385) -> (-964562.8938, -606554.1144)
  line L569 (-964562.8938, -606554.1144) -> (-956331.8926, -563335.7128)
  line L570 (-956331.8926, -563335.7128) -> (-756273.4332, -588744.7369)
  line L571 (-756273.4332, -588744.7369) -> (-764504.4344, -631963.1385)
  line L572 (-775108.3703, -687641.0747) -> (-768853.0044, -654796.1136)
  line L573 (-768853.0044, -654796.1136) -> (-853304.0886, -638712.294)
  line L574 (-853304.0886, -638712.294) -> (-858178.4293, -677090.5129)
  line L575 (-858178.4293, -677090.5129) -> (-775108.3703, -687641.0747)
  line L576 (-878747.9475, -671938.5981) -> (-874181.048, -635981.0233)
  line L577 (-874181.048, -635981.0233) -> (-949276.209, -621679.0516)
  line L578 (-949276.209, -621679.0516) -> (-953559.2883, -644168.1558)
  line L579 (-953559.2883, -644168.1558) -> (-878747.9475, -671938.5981)
  line L580 (-447334.3793, -416555.467) -> (-478627.8111, -448739.9886)
  line L581 (-478627.8111, -448739.9886) -> (-495178.3039, -432647.7278)
  line L582 (-495178.3039, -432647.7278) -> (-450129.7444, -407055.8814)
  line L583 (-450129.7444, -407055.8814) -> (-447334.3793, -416555.467)
  line L584 (-513487.4448, -583577.8917) -> (-510927.7536, -563424.1118)
  line L585 (-510927.7536, -563424.1118) -> (-518906.7224, -562410.719)
  line L586 (-518906.7224, -562410.719) -> (-518634.5613, -558855.9891)
  line L587 (-518634.5613, -558855.9891) -> (-526115.9628, -557905.7913)
  line L588 (-526115.9628, -557905.7913) -> (-529124.2865, -581591.8878)
  line L589 (-529124.2865, -581591.8878) -> (-513487.4448, -583577.8917)
  line L590 (-422565.3067, -361435.3408) -> (-413989.3518, -306980.1936)
  line L591 (-413989.3518, -306980.1936) -> (-487373.0762, -298546.9503)
  line L592 (-487373.0762, -298546.9503) -> (-488784.1843, -307507.1304)
  line L593 (-488784.1843, -307507.1304) -> (-421939.4296, -318034.2822)
  line L594 (-421939.4296, -318034.2822) -> (-430038.0568, -361435.3408)
  line L595 (-430038.0568, -361435.3408) -> (-422565.3067, -361435.3408)
  line L596 (-426890.2142, -388897.411) -> (-499793.9023, -377416.0586)
  line L597 (-499793.9023, -377416.0586) -> (-499651.4672, -376511.6316)
  line L598 (-499651.4672, -376511.6316) -> (-494518.3408, -368976.445)
  line L599 (-494518.3408, -368976.445) -> (-425465.5776, -379851.3285)
  line L600 (-425465.5776, -379851.3285) -> (-426890.2142, -388897.411)
  line L601 (-239023.3878, -418109.7481) -> (-391233.048, -394138.7694)
  line L602 (-391233.048, -394138.7694) -> (-389865.9115, -385457.7981)
  line L603 (-389865.9115, -385457.7981) -> (-233550.2353, -410075.4193)
  line L604 (-233550.2353, -410075.4193) -> (-239023.3878, -418109.7481)
  line L605 (-144108.783, -303905.1502) -> (-138961.9977, -271224.3636)
  line L606 (-138961.9977, -271224.3636) -> (-179720.8947, -264805.3844)
  line L607 (-179720.8947, -264805.3844) -> (-184564.7198, -295562.4501)
  line L608 (-184564.7198, -295562.4501) -> (-143805.8228, -301981.4294)
  line L609 (-143805.8228, -301981.4294) -> (-143736.749, -301542.8279)
  line L610 (-156664.9556, -377175.143) -> (-180340.0287, -368452.1025)
  line L611 (-180340.0287, -368452.1025) -> (-180340.0287, -357474.5668)
  line L612 (-180340.0287, -357474.5668) -> (-151068.1018, -357474.5668)
  line L613 (-156664.9556, -377175.143) -> (-151068.1018, -357474.5668)
  line L614 (-160965.2, -430402.8651) -> (-205892.2219, -423327.4621)
  line L615 (-205892.2219, -423327.4621) -> (-200065.7498, -386330.836)
  line L616 (-200065.7498, -386330.836) -> (-158319.3671, -394138.7694)
  line L617 (-158319.3671, -394138.7694) -> (-160965.2, -430402.8651)
  line L618 (-118476.5784, -429084.8633) -> (-118476.5784, -326152.1723)
  line L619 (-118476.5784, -326152.1723) -> (-142169.5365, -326152.1723)
  line L620 (-142169.5365, -326152.1723) -> (-149259.4577, -423327.4621)
  line L621 (-149259.4577, -423327.4621) -> (-118476.5784, -429084.8633)
  point P0 (0, 0)
  point P1 (-134865.3071, -753610.3454)
  dimension "d1" = 1275000
  constraints: 1236 end point, 282 perpendicular, 183 point on line, 136 parallel, 11 vertical, 8 horizontal, 3 collinear, 1 midpoint, 2 other
  measures "d1" distance between parallel lines of L3 L1